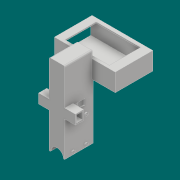
# Autodesk Inventor part: InternalSupport
Saved by Autodesk Inventor 2017.3 (Build 213257000, 257)
## iProperties
Created: 2019-12-07
Part Number: InternalSupport
Material: Generic
Document SubType Name: Modeling
Designer: Santiago
Density: 1 g/cm^3
Appearance: Default
Author: Santiago
Autodesk Inventor part; units mm, degrees
ref_plane "YZ Plane" through (0, 0, 0) normal (1, 0, 0) x (0, 1, 0)
ref_plane "XZ Plane" through (0, 0, 0) normal (0, 1, 0) x (-1, 0, 0)
ref_plane "XY Plane" through (0, 0, 0) normal (0, 0, 1) x (1, 0, 0)
sketch "Sketch1" plane through (0, 0, 0) normal (0, 0, 1) x (1, 0, 0)
  line L0 (0, 0) -> (22, 0)
  line L1 (22, 0) -> (22, 45)
  line L2 (22, 45) -> (0, 45)
  line L3 (0, 45) -> (0, 0)
  line L4 (-2, 47) -> (24, 47)
  line L5 (24, 47) -> (24, -2)
  line L6 (24, -2) -> (-2, -2)
  line L7 (-2, -2) -> (-2, 47)
  dimension "d0" = 22
  dimension "d1" = 45
  dimension "d2" = 2
  constraints: 16 end point, 4 perpendicular, 1 horizontal, 1 vertical, 3 other
  measures "d0" distance of L0.start L0.end
  measures "d1" distance of L0.end L1.end
  measures "d2" distance between parallel lines of L2 L4
extrude "Extrusion1" add sketch "Sketch1" along normal blind 40
sketch "Sketch2" plane through (24, -2, 0) normal (1, 0, 0) x (0, 0, -1)
  line L0 (0, 0) -> (-40, 0) projected
  line L1 (-20, 0) -> (-20, 2)
  line L2 (-20, 2) -> (-14, 2)
  line L3 (-14, 2) -> (-14, 12)
  line L4 (-14, 12) -> (-26, 12)
  line L5 (-26, 12) -> (-26, 2)
  line L6 (-26, 2) -> (-14, 2)
  line L7 (-28, 14) -> (-12, 14)
  line L8 (-12, 14) -> (-12, 0)
  line L9 (-12, 0) -> (-28, 0)
  line L10 (-28, 0) -> (-28, 14)
  point P0 (0, 2)
  dimension "d5" = 2
  dimension "d6" = 6
  dimension "d7" = 10
  dimension "d8" = 12
  dimension "d9" = 2
  constraints: 20 end point, 6 perpendicular, 1 midpoint, 1 parallel, 1 point on line, 1 vertical, 3 other
  measures "d5" distance of L1.start L1.end
  measures "d6" distance of L1.end L2.end
  measures "d7" distance of L2.end L3.end
  measures "d8" distance of L3.end L4.end
  measures "d9" distance between parallel lines of L4 L7
extrude "Extrusion2" add sketch "Sketch2" along normal blind 18
sketch "Sketch3" plane through (-2, -2, 0) normal (-1, 0, 0) x (0, 0, 1)
  line L0 (26, 12) -> (26, 2) projected
  line L1 (14, 12) -> (26, 12) projected
  line L2 (14, 2) -> (14, 12) projected
  line L3 (0, 2) -> (40, 2) projected
  line L4 (28, 0) -> (28, 14) projected
  line L5 (28, 14) -> (12, 14) projected
  line L6 (12, 14) -> (12, 0) projected
  line L7 (0, 0) -> (40, 0) projected
extrude "Extrusion3" add sketch "Sketch3" along normal blind 18 contours L1 L2 L3 L6 L5 L4 L0 | L3 L4 L7 L6
sketch "Sketch4" plane through (-2, 0, 26) normal (-1, 0, 0) x (0, 0, 1)
  line L0 (-12, 0) -> (0, 0) projected
  line L1 (0, 0) -> (0, 10) projected
  line L2 (0, 10) -> (-12, 10) projected
  line L3 (-12, 10) -> (-12, 0) projected
  point P0 (-26, 0)
extrude "Extrusion4" cut sketch "Sketch4" against normal blind 40
sketch "Sketch5" plane through (24, 12, 28) normal (0, 1, 0) x (1, 0, 0)
  line L0 (-26, 28) -> (-26, -12) projected
  line L1 (0, 28) -> (0, -12) projected
  line L2 (0, 8) -> (0, 13)
  line L3 (0, 13) -> (0, 3)
  line L4 (0, 13) -> (-2, 13)
  line L5 (-2, 13) -> (-2, 3)
  line L6 (-2, 28) -> (-2, -12) projected
  line L7 (-2, 3) -> (0, 3)
  line L8 (0, 3) -> (5, 3)
  line L9 (5, 3) -> (5, 13)
  line L10 (5, 13) -> (0, 13)
  line L11 (-26, 28) -> (0, 28) projected
  line L12 (-13, 28) -> (-13, 3)
  line L13 (-26, 28) -> (-26, -12)
  line L14 (-26, 8) -> (-26, 13)
  line L15 (-26, 13) -> (-26, 3)
  line L16 (-26, 13) -> (-24, 13)
  line L17 (-24, 13) -> (-24, 3)
  line L18 (-24, 28) -> (-24, -12)
  line L19 (-24, 3) -> (-26, 3)
  line L20 (-26, 3) -> (-31, 3)
  line L21 (-31, 3) -> (-31, 13)
  line L22 (-31, 13) -> (-26, 13)
  dimension "d16" = 5
  dimension "d17" = 10
  dimension "d18" = 2
  dimension "d19" = 5
  constraints: 38 end point, 10 point on line, 8 symmetric about line, 3 perpendicular, 2 midpoint, 1 horizontal, 1 vertical
  measures "d16" distance of L2.start L2.end
  measures "d17" distance of L2.end L3.end
  measures "d18" distance of L2.end L4.end
  measures "d19" distance of L3.end L8.end
extrude "Extrusion5" cut sketch "Sketch5" along normal blind 20 contours L16 L17 L19 L0 | L0 L20 L21 L22 | L4 L1 L7 L5 | L10 L9 L8 L1
sketch "Sketch6" plane through (-20, 12, 12) normal (0, 1, 0) x (1, 0, 0)
  line L0 (20, -3) -> (18, -3) projected
  line L1 (18, -13) -> (20, -13) projected
  line L2 (20, -3) -> (20, -13) projected
  line L3 (42, -13) -> (42, -3) projected
  line L4 (44, -3) -> (42, -3) projected
  line L5 (42, -13) -> (44, -13) projected
  line L6 (44, -3) -> (44, 0) projected
  line L7 (44, -3) -> (44, -13)
  line L8 (18, -3) -> (18, -13)
  line L9 (18, -13) -> (13, -13)
  line L10 (13, -13) -> (13, -3)
  line L11 (13, -3) -> (18, -3)
  line L12 (44, -16) -> (44, -13) projected
  line L13 (44, -13) -> (49, -13)
  line L14 (49, -13) -> (49, -3)
  line L15 (49, -3) -> (44, -3)
  line L16 (44, -13) -> (44, -3)
  point P0 (20, 12)
  dimension "d22" = 5
  dimension "d23" = 5
  constraints: 18 end point, 4 perpendicular, 2 point on line, 1 collinear, 1 horizontal, 1 parallel, 1 vertical
  measures "d22" distance of L1.start L9.end
  measures "d23" distance of L5.end L13.end
extrude "Extrusion6" cut sketch "Sketch6" against normal blind 5
sketch "Sketch7" plane through (0, 0, 40) normal (0, 0, 1) x (1, 0, 0)
  line L0 (0, 0) -> (0, 45) projected
  line L1 (0, 45) -> (22, 45) projected
  line L2 (22, 45) -> (22, 0) projected
  line L3 (22, 0) -> (0, 0) projected
  line L4 (24, 47) -> (-2, 47) projected
  line L5 (-2, 47) -> (-2, -2) projected
  line L6 (-2, -2) -> (24, -2) projected
  line L7 (24, -2) -> (24, 47) projected
extrude "Extrusion7" add sketch "Sketch7" along normal blind 30
sketch "Sketch8" plane through (0, 0, 0) normal (0, 0, -1) x (-1, 0, 0)
  line L0 (-22, 45) -> (0, 45) projected
  line L1 (-22, 44) -> (0, 44)
  line L2 (-22, 44) -> (-22, 45)
  line L3 (2, 47) -> (-24, 47) projected
  line L4 (0, 0) -> (0, 45) projected
  line L5 (0, 44) -> (0, 45)
  line L6 (0, 45) -> (-22, 45) projected
  line L7 (0, 45) -> (-22, 45)
  dimension "d28" = 1
  constraints: 8 end point, 2 perpendicular, 1 parallel, 1 vertical
  measures "d28" distance between parallel lines of L0 L1
extrude "Extrusion8" add sketch "Sketch8" against normal blind 70
sketch "Sketch9" plane through (-2, 47, 0) normal (0, 1, 0) x (1, 0, 0)
  line L0 (0, 0) -> (26, 0) projected
  line L1 (0, 0) -> (0, -70) projected
  line L2 (26, -70) -> (0, -70) projected
  line L3 (26, 0) -> (26, -70) projected
  point P0 (2, 0)
extrude "Extrusion9" cut sketch "Sketch9" against normal blind 1
sketch "Sketch10" plane through (0, 0, 70) normal (0, 0, 1) x (1, 0, 0)
  line L0 (24, 46) -> (-2, 46) projected
  line L1 (-2, 46) -> (-2, -2) projected
  line L2 (-2, -2) -> (24, -2) projected
  line L3 (24, -2) -> (24, 46) projected
  line L4 (22, 44) -> (22, 0) projected
  line L5 (22, 0) -> (0, 0) projected
  line L6 (0, 0) -> (0, 44) projected
  line L7 (0, 44) -> (22, 44) projected
extrude "Extrusion10" add sketch "Sketch10" along normal blind 17.25
sketch "Sketch11" plane through (0, 0, 0) normal (0, 0, -1) x (-1, 0, 0)
  line L0 (2, 46) -> (-24, 46) projected
  line L1 (-24, 46) -> (-24, -2) projected
  line L2 (-24, -2) -> (2, -2) projected
  line L3 (2, -2) -> (2, 46) projected
  line L4 (0, 44) -> (0, 0) projected
  line L5 (0, 0) -> (-22, 0) projected
  line L6 (-22, 0) -> (-22, 44) projected
  line L7 (0, 44) -> (-22, 44) projected
extrude "Extrusion11" add sketch "Sketch11" along normal blind 47.25
sketch "Sketch12" plane through (24, -2, 28) normal (1, 0, 0) x (0, 0, -1)
  circle A0 centre (70.3128, 35.4495) radius 0.5
  line L0 (70.3128, 35.4495) -> (70.3128, 13.6495)
  circle A1 centre (70.3128, 13.6495) radius 0.5
  line L1 (70.3128, 35.4495) -> (26.0128, 35.4495)
  line L2 (26.0128, 35.4495) -> (26.0128, 13.6495)
  circle A2 centre (26.0128, 35.4495) radius 0.5
  circle A3 centre (26.0128, 13.6495) radius 0.5
  circle A4 centre (26.0128, 35.4495) radius 2.5
  circle A5 centre (26.0128, 13.6495) radius 2.5
  circle A6 centre (70.3128, 35.4495) radius 2.5
  circle A7 centre (70.3128, 13.6495) radius 2.5
  point P0 (28, 2)
  dimension "d37" = 1
  dimension "d38" = 21.8
  dimension "d39" = 1
  dimension "d40" = 44.3
  dimension "d41" = 1
  dimension "d42" = 1
  dimension "d43" = 2
  dimension "d44" = 2
  dimension "d45" = 2
  dimension "d46" = 2
  constraints: 8 centre point, 6 end point, 3 coincident, 1 horizontal, 1 perpendicular, 1 vertical
  measures "d37" diameter of A0
  measures "d38" distance of L0.start L0.end
  measures "d39" diameter of A1
  measures "d40" distance of L0.start L1.end
  measures "d41" diameter of A2
  measures "d42" diameter of A3
  measures "d43" radial gap between concentric circles of A2 A4
  measures "d44" radial gap between concentric circles of A3 A5
  measures "d45" radial gap between concentric circles of A0 A6
  measures "d46" radial gap between concentric circles of A1 A7
extrude "Extrusion12" add sketch "Sketch12" along normal blind 2 contours A0 L1 A6 L0 | A0 L0 A6 L1 | A5 | A4 L2 A2 L1 | L1 A2 L2 A4 | A7
sketch "Sketch13" plane through (-2, 46, 0) normal (0, 1, 0) x (1, 0, 0)
  line L0 (0, -87.25) -> (0, 47.25) projected
  line L1 (0, -20) -> (0, 2)
  line L2 (0, 2) -> (0, -42)
  line L3 (0, 2) -> (26, 2)
  line L4 (26, 47.25) -> (26, -87.25) projected
  line L5 (13, 2) -> (-9, 2)
  line L6 (-9, 2) -> (-9, -42)
  line L7 (-9, -42) -> (35, -42)
  line L8 (35, -42) -> (35, 2)
  line L9 (35, 2) -> (-9, 2)
  point P0 (2, 0)
  dimension "d49" = 22
  dimension "d50" = 44
  dimension "d51" = 22
  dimension "d52" = 44
  dimension "d53" = 44
  constraints: 16 end point, 4 point on line, 3 perpendicular, 2 horizontal, 2 midpoint, 1 collinear
  measures "d49" distance of L1.start L1.end
  measures "d50" distance of L1.end L2.end
  measures "d51" distance of L5.start L5.end
  measures "d52" distance of L5.end L6.end
  measures "d53" distance of L6.end L7.end
extrude "Extrusion13" add sketch "Sketch13" against normal blind 2
sketch "Sketch14" plane through (-2, 46, 0) normal (0, 1, 0) x (1, 0, 0)
  line L0 (35, 2) -> (35, -42) projected
  line L1 (35, 2) -> (35, -1.5)
  line L2 (35, -1.5) -> (31.5, -1.5)
  circle A0 centre (31.5, -1.5) radius 1
  line L3 (35, -20) -> (25.0938, -20)
  circle A1 centre (31.5, -38.5) radius 1
  line L4 (2, 47.25) -> (24, 47.25) projected
  line L5 (13, 47.25) -> (13, 21.5111)
  circle A2 centre (-5.5, -1.5) radius 1
  circle A3 centre (-5.5, -38.5) radius 1
  circle A4 centre (-5.5, -38.5) radius 2
  circle A5 centre (-5.5, -1.5) radius 2
  circle A6 centre (31.5, -38.5) radius 2
  circle A7 centre (31.5, -1.5) radius 2
  point P0 (2, 0)
  dimension "d56" = 3.5
  dimension "d57" = 3.5
  dimension "d58" = 2
  dimension "d59" = 1
  dimension "d60" = 1
  dimension "d61" = 1
  dimension "d62" = 1
  constraints: 8 centre point, 8 end point, 3 symmetric about line, 2 midpoint, 1 coincident, 1 horizontal, 1 perpendicular, 1 point on line, 1 vertical, 3 other
  measures "d56" distance of L0.start L1.end
  measures "d57" distance of L1.end L2.end
  measures "d58" diameter of A0
  measures "d59" radial gap between concentric circles of A3 A4
  measures "d60" radial gap between concentric circles of A2 A5
  measures "d61" radial gap between concentric circles of A1 A6
  measures "d62" radial gap between concentric circles of A0 A7
extrude "Extrusion14" add sketch "Sketch14" along normal blind 1
sketch "Sketch15" plane through (-2, 46, 0) normal (0, 1, 0) x (1, 0, 0)
  circle A0 centre (-5.5, -38.5) radius 1 projected
  circle A1 centre (-5.5, -1.5) radius 1 projected
  circle A2 centre (31.5, -1.5) radius 1 projected
  circle A3 centre (31.5, -38.5) radius 1 projected
  point P0 (2, 0)
extrude "Extrusion15" cut sketch "Sketch15" against normal blind 3
sketch "Sketch16" plane through (-2, 46, 0) normal (0, 1, 0) x (1, 0, 0)
  line L0 (24, -87.25) -> (24, 47.25) projected
  line L1 (2, 47.25) -> (2, -87.25) projected
  line L2 (2, -14) -> (2, 47.25) projected
  line L3 (2, 47.25) -> (2, -2.75)
  line L4 (2.012, -37.9877) -> (4.512, -37.9877)
  circle A0 centre (4.512, -37.9877) radius 1
  line L5 (4.512, -37.9877) -> (4.512, -67.9877)
  line L6 (4.5, -37.75) -> (21, -37.75)
  circle A1 centre (20.988, -7.5123) radius 1
  circle A2 centre (4.512, -37.9877) radius 2
  circle A3 centre (20.988, -7.5123) radius 2
  line L7 (21, -7.75) -> (21, -37.75)
  point P0 (2, 0)
  dimension "d67" = 50
  dimension "d68" = 2.5
  dimension "d69" = 2
  dimension "d70" = 30
  dimension "d71" = 16.5
  dimension "d72" = 2
  dimension "d73" = 1
  dimension "d74" = 1
  dimension "d91" = 30
  constraints: 10 end point, 4 centre point, 2 perpendicular, 1 coincident, 1 parallel
  measures "d67" distance of L3.end L1.start
  measures "d68" distance of L4.start L4.end
  measures "d69" diameter of A0
  measures "d70" distance of L5.end L5.start
  measures "d71" distance of L6.start L6.end
  measures "d72" diameter of A1
  measures "d73" radial gap between concentric circles of A0 A2
  measures "d74" radial gap between concentric circles of A1 A3
  measures "d91" distance of L7.start L7.end
extrude "Extrusion16" add sketch "Sketch16" along normal blind 1 contours A2 L6 A0 L4 | A3 | L4 A0 L5 A2 | A2 L5 A0 L6
sketch "Sketch17" plane through (-2, 46, 0) normal (0, 1, 0) x (1, 0, 0)
  circle A0 centre (4.512, -37.9877) radius 1 projected
  circle A1 centre (20.988, -7.5123) radius 1 projected
  point P0 (2, 0)
extrude "Extrusion17" cut sketch "Sketch17" against normal blind 3
sketch "Sketch18" plane through (-2, 46, 0) normal (0, 1, 0) x (1, 0, 0)
  line L0 (-9, -42) -> (0, -42) projected
  line L1 (0, -87.25) -> (0, -42) projected
  line L2 (0, -47) -> (26, -47)
  line L3 (26, -42) -> (26, -87.25) projected
  line L4 (0, -49) -> (26, -49)
  line L5 (0, -75) -> (26, -75)
  line L6 (0, -77) -> (26, -77)
  line L7 (0, -47) -> (0, -49)
  line L8 (26, -47) -> (26, -49)
  line L9 (26, -75) -> (26, -77)
  line L10 (0, -75) -> (0, -77)
  point P0 (2, 0)
  dimension "d79" = 5
  dimension "d80" = 2
  dimension "d81" = 26
  dimension "d82" = 2
  constraints: 16 end point, 4 parallel, 2 collinear, 2 point on line, 1 perpendicular
  measures "d79" distance of L0.end L2.start
  measures "d80" distance between parallel lines of L2 L4
  measures "d81" distance between parallel lines of L4 L5
  measures "d82" distance between parallel lines of L5 L6
extrude "Extrusion18" add sketch "Sketch18" along normal blind 30 contours L1 L2 L3 L4
sketch "Sketch19" plane through (-2, 46, 0) normal (0, 1, 0) x (1, 0, 0)
  line L0 (0, -49) -> (26, -49) projected
  line L1 (0, -75) -> (26, -75)
  line L2 (0, -77) -> (26, -77)
  line L3 (0, -75) -> (0, -77)
  line L4 (0, -28) -> (0, -87.25) projected
  line L5 (26, -75) -> (26, -77)
  line L6 (26, -49) -> (26, -87.25) projected
  point P0 (2, 0)
  dimension "d85" = 26
  dimension "d86" = 2
  constraints: 8 end point, 2 collinear, 2 parallel
  measures "d85" distance between parallel lines of L0 L1
  measures "d86" distance between parallel lines of L1 L2
extrude "Extrusion19" add sketch "Sketch19" along normal blind 3 contours L1 L5 L2 L3
sketch "Sketch20" plane through (-2, 46, 0) normal (0, 1, 0) x (1, 0, 0)
  line L0 (26, -42) -> (26, -47) projected
  line L1 (26, 47.25) -> (26, 2) projected
  line L2 (0, 2) -> (0, 47.25) projected
  line L3 (0, -47) -> (0, -42) projected
  line L4 (26, -42) -> (26, 2)
  line L5 (35, -42) -> (35, 2) projected
  line L6 (35, 2) -> (26, 2) projected
  line L7 (26, -42) -> (35, -42) projected
  line L8 (-9, 2) -> (-9, -42) projected
  line L9 (-9, -42) -> (0, -42) projected
  line L10 (0, 2) -> (-9, 2) projected
  line L11 (0, -42) -> (0, 2) projected
  point P0 (2, 0)
  constraints: 2 end point, 1 collinear
extrude "Extrusion20" cut sketch "Sketch20" along normal mid plane 10
sketch "Sketch21" plane through (-2, 46, 0) normal (0, 1, 0) x (1, 0, 0)
  line L0 (0, 47.25) -> (26, 47.25) projected
  line L1 (24, -87.25) -> (24, 47.25) projected
  line L2 (2, 47.25) -> (2, -87.25) projected
  line L3 (26, 47.25) -> (0, 47.25) projected
  circle A0 centre (13, 47.25) radius 11
  point P0 (2, 0)
  constraints: 1 horizontal alignment, 1 midpoint, 2 other
extrude "Extrusion21" cut sketch "Sketch21" against normal blind 100
sketch "Sketch22" plane through (0, 0, 87.25) normal (0, 0, 1) x (1, 0, 0)
  line L0 (22, 0) -> (0, 0) projected
  line L1 (0, 0) -> (0, 44) projected
  line L2 (0, 44) -> (22, 44) projected
  line L3 (22, 44) -> (22, 0) projected
  line L4 (24, 46) -> (-2, 46) projected
  line L5 (-2, 46) -> (-2, -2) projected
  line L6 (-2, -2) -> (24, -2) projected
  line L7 (24, -2) -> (24, 46) projected
extrude "Extrusion22" add sketch "Sketch22" along normal blind 2 contours L0 L1 L2 L3 | L7 L6 L5 L4
sketch "Sketch24" plane through (-2, 46, 77) normal (0, 0, 1) x (1, 0, 0)
  line L0 (0, 3) -> (26, 3) projected
  line L1 (26, 3) -> (0, 3) projected
  line L2 (13, 3) -> (50.3, 3)
  line L3 (50.3, 3) -> (-24.3, 3)
  line L4 (-24.3, 3) -> (-24.3, 0)
  line L5 (-24.3, 0) -> (50.3, 0)
  line L6 (50.3, 0) -> (50.3, 3)
  point P0 (2, -46)
  dimension "d98" = 37.3
  dimension "d99" = 74.6
  dimension "d100" = 3
  constraints: 10 end point, 3 perpendicular, 2 point on line, 1 midpoint
  measures "d98" distance of L2.start L2.end
  measures "d99" distance of L2.end L3.end
  measures "d100" distance of L3.end L4.end
extrude "Extrusion24" add sketch "Sketch24" against normal blind 2
sketch "Sketch25" plane through (24, 46, 77) normal (0, 0, 1) x (1, 0, 0)
  line L0 (-50.3, 0) -> (-50.3, 3) projected
  line L1 (-50.3, 0) -> (-63.3, 0)
  line L2 (24.3, 0) -> (0, 0) projected
  line L3 (24.3, 0) -> (37.3, 0)
  line L4 (24.3, 57.5) -> (-50.3, 57.5)
  line L5 (-63.3, 57.5) -> (-63.3, 0)
  line L6 (-50.3, 3) -> (24.3, 3) projected
  line L7 (-50.3, 3) -> (-50.3, 57.5)
  line L8 (24.3, 3) -> (24.3, 57.5)
  line L9 (-63.3, 57.5) -> (-63.3, 59.5)
  line L10 (-63.3, 59.5) -> (37.3, 59.5)
  line L11 (37.3, 0) -> (37.3, 57.5)
  line L12 (37.3, 57.5) -> (37.3, 59.5)
  line L13 (37.3, 59.5) -> (-63.3, 59.5)
  line L14 (-63.3, 0) -> (-50.3, 0)
  line L15 (-26, 0) -> (-50.3, 0) projected
  line L16 (-50.3, 3) -> (-50.3, 0)
  line L17 (24.3, 3) -> (24.3, 0)
  line L18 (37.3, 0) -> (24.3, 0)
  line L19 (24.3, 57.5) -> (24.3, 0)
  point P0 (-24, -46)
  dimension "d103" = 13
  dimension "d104" = 13
  dimension "d105" = 57.5
  dimension "d106" = 2
  dimension "d107" = 57.5
  dimension "d108" = 2
  constraints: 32 end point, 4 perpendicular, 4 vertical, 3 collinear, 2 horizontal, 2 parallel
  measures "d103" distance of L0.start L1.end
  measures "d104" distance of L2.start L3.end
  measures "d105" distance of L3.end L11.end
  measures "d106" distance of L5.start L9.end
  measures "d107" distance of L3.end L11.end
  measures "d108" distance of L11.end L10.end
extrude "Extrusion25" add sketch "Sketch25" against normal blind 2 contours L1 L5 L9 L10 L12 L11 L3 L17 L8 L4 L7 L0
sketch "Sketch26" plane through (24, 46, 75) normal (0, -1, 0) x (1, 0, 0)
  line L0 (0, 0) -> (0, 2) projected
  line L1 (37.3, 0) -> (0, 0) projected
  line L2 (37.3, 2) -> (37.3, 0) projected
  line L3 (0, 2) -> (37.3, 2) projected
  line L4 (0, 0) -> (0, 2) projected
  line L5 (0, 2) -> (0, -28)
  line L6 (0, -28) -> (37.3, -28)
  line L7 (37.3, -28) -> (37.3, 2)
  point P0 (-24, -75)
  constraints: 6 end point, 1 parallel, 1 perpendicular, 1 vertical
extrude "Extrusion26" add sketch "Sketch26" along normal blind 2
sketch "Sketch27" plane through (-2, 46, 0) normal (0, 1, 0) x (1, 0, 0)
  line L0 (0, -75) -> (0, -49) projected
  line L1 (-37.3, -75) -> (63.3, -75) projected
  line L2 (0, -77) -> (0, -75) projected
  line L3 (0, -77) -> (-37.3, -77) projected
  line L4 (-37.3, -77) -> (-37.3, -75) projected
  line L5 (0, -75) -> (-37.3, -75) projected
  line L6 (-37.3, -77) -> (-37.3, -49)
  line L7 (26, -49) -> (0, -49) projected
  line L8 (-37.3, -49) -> (0, -49)
  line L9 (0, -49) -> (0, -75)
  line L10 (63.3, -77) -> (-37.3, -77) projected
  line L11 (26, -77) -> (0, -77) projected
  line L12 (-37.3, -77) -> (0, -77)
  line L13 (0, -77) -> (0, -49)
  line L14 (0, -49) -> (0, -47)
  line L15 (0, -28) -> (0, -89.25) projected
  line L16 (0, -47) -> (-37.3, -47)
  line L17 (-37.3, -47) -> (-37.3, -49)
  point P0 (2, 0)
  dimension "d113" = 2
  constraints: 16 end point, 4 perpendicular, 1 collinear, 1 horizontal, 1 point on line, 1 vertical
  measures "d113" distance of L0.end L14.end
extrude "Extrusion27" add sketch "Sketch27" against normal blind 2
sketch "Sketch28" plane through (-2, 46, 77) normal (0, 0, 1) x (1, 0, 0)
  line L0 (-24.3, 57.5) -> (50.3, 57.5) projected
  line L1 (-24.3, 55.5) -> (50.3, 55.5)
  line L2 (-24.3, 57.5) -> (-24.3, 3) projected
  line L3 (-24.3, 55.5) -> (-24.3, 57.5)
  line L4 (-24.3, 57.5) -> (50.3, 57.5)
  line L5 (50.3, 3) -> (50.3, 57.5) projected
  line L6 (50.3, 55.5) -> (50.3, 57.5)
  point P0 (2, -46)
  dimension "d116" = 2
  constraints: 8 end point, 2 collinear, 1 parallel, 1 vertical
  measures "d116" distance between parallel lines of L0 L1
extrude "Extrusion28" add sketch "Sketch28" against normal blind 2
sketch "Sketch29" plane through (-39.3, 105.5, 77) normal (0, 1, 0) x (1, 0, 0)
  line L0 (100.6, 0) -> (0, 0) projected
  line L1 (100.6, 0) -> (100.6, 2) projected
  line L2 (0, 2) -> (100.6, 2) projected
  line L3 (0, 0) -> (0, 2) projected
  line L4 (63.3, 30) -> (37.3, 30) projected
  line L5 (37.3, 30) -> (37.3, 28) projected
  line L6 (37.3, 28) -> (63.3, 28) projected
  line L7 (63.3, 28) -> (63.3, 30) projected
  line L8 (63.3, 30) -> (100.6, 30) projected
  line L9 (100.6, 0) -> (100.6, 30)
  line L10 (100.6, 30) -> (0, 30)
  line L11 (0, 30) -> (0, 0)
  point P0 (39.3, 77)
  constraints: 6 end point, 2 perpendicular, 1 vertical
extrude "Extrusion29" add sketch "Sketch29" along normal blind 2
sketch "Sketch30" plane through (61.3, 46, 75) normal (1, 0, 0) x (0, 0, -1)
  line L0 (-2, 61.5) -> (28, 61.5) projected
  line L1 (-2, -2) -> (-2, 61.5) projected
  line L2 (28, -2) -> (-2, -2) projected
  line L3 (28, 0) -> (28, 30) projected
  line L4 (28, 0) -> (28, -2) projected
  line L5 (28, 59.5) -> (28, 61.5) projected
  line L6 (28, 61.5) -> (28, 30)
  point P0 (75, -46)
  constraints: 2 end point, 1 collinear
extrude "Extrusion30" add sketch "Sketch30" along normal blind 2
sketch "Sketch31" plane through (61.3, 105.5, 47) normal (0, 0, -1) x (-1, 0, 0)
  line L0 (100.6, 2) -> (-2, 2) projected
  line L1 (-2, -61.5) -> (-2, 2) projected
  line L2 (37.3, -61.5) -> (-2, -61.5) projected
  line L3 (100.6, -61.5) -> (63.3, -61.5) projected
  line L4 (100.6, -59.5) -> (100.6, 0) projected
  line L5 (100.6, -59.5) -> (100.6, -61.5) projected
  line L6 (100.6, 0) -> (100.6, 2) projected
  line L7 (37.3, -61.5) -> (63.3, -61.5)
  point P0 (61.3, -105.5)
  constraints: 2 end point, 1 horizontal
extrude "Extrusion31" add sketch "Sketch31" against normal blind 2
fillet "Fillet1" radius 2 2 edges at (-2, 22, 89.25) (24, 22, 89.25)
fillet "Fillet2" radius 2 3 edges at (-2, 46, -0.125) (24, 46, -0.125) (11, 46, 89.25)
body "Solid1"
